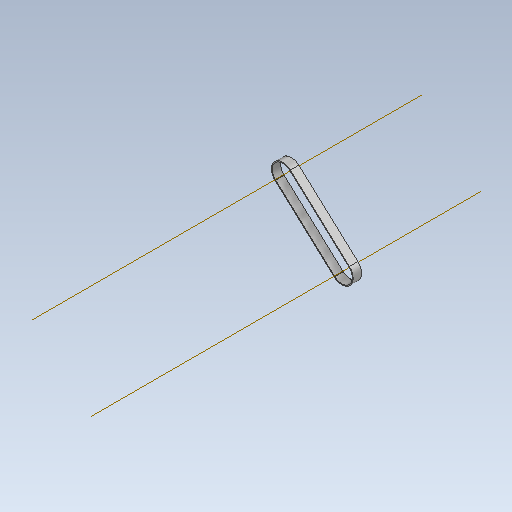
# Autodesk Inventor part: Synchronous Belt
Saved by Autodesk Inventor 2020 (Build 240168000, 168)
## iProperties
Created: 2022-07-06
Part Number: Synchronous Belt
Material: Rubber
Document SubType Name: Modeling
Designer: karimi2
Density: 1 g/cm^3
Appearance: Rubber - Black - Version 1.1
CustomPartVersion: 1
Author: karimi2
Autodesk Inventor part; units mm, degrees
sketch "Sketch Path" plane through (0, 0, 0) normal (0, 0, 1) x (1, 0, 0)
  arc A0 (-122.9906, 123.6577) -> (-133.8904, 111.7133) centre (-128.4405, 117.6855) ccw
  arc A1 (-89.5701, 71.2694) -> (-78.6704, 83.2138) centre (-84.1202, 77.2416) ccw
  line L0 (-89.5701, 71.2694) -> (-133.8904, 111.7133)
  line L1 (-122.9906, 123.6577) -> (-78.6704, 83.2138)
  constraints: 4 end point, 4 point on circle, 2 centre point
ref_plane "Cross Section Plane" through (-133.8904, 111.7133, 0) normal (0.7387, -0.6741, 0) x (0, 0, 1)
ref_plane "Work Plane2" through (-128.4405, 117.6855, 0) normal (-1, 0, 0) x (0, 0, 1)
ref_plane "Work Plane3" through (-84.1202, 77.2416, 0) normal (-0.6427, 0.7661, 0) x (0, 0, 1)
sketch "Cross Section" plane through (-133.8904, 111.7133, 0) normal (0.7387, -0.6741, 0) x (0, 0, 1)
  line L0 (-3.175, 0.381) -> (3.175, 0.381)
  line L1 (3.175, 0.381) -> (3.175, -0.254)
  line L2 (3.175, -0.254) -> (-3.175, -0.254)
  line L3 (-3.175, -0.254) -> (-3.175, 0.381)
  line L4 (-3.175, 0) -> (3.175, 0) construction
  point P0 (0, 0)
  point P1 (0, 0)
  dimension "d0" = 6.35
  dimension "d4" = 0.254
  dimension "d5" = 0.381
  constraints: 10 end point, 2 parallel, 2 point on line, 1 coincident, 1 horizontal, 1 midpoint, 1 perpendicular, 1 other
  measures "d0" distance between parallel lines of L1 L3
  measures "d4" distance between parallel lines of L2 L4
  measures "d5" distance between parallel lines of L4 L0
sweep "Belt" add profiles "Cross Section" path "Sketch Path"
equation "\"d0\" = da_B"
equation "\"d4\" = da_a"
equation "\"d5\" = da_a2"
equation "\"da_B\" = 6.35"
equation "\"da_pb\" = 2.032"
equation "\"da_L\" = 170.8"
equation "\"da_a\" = 0.254"
equation "\"da_S\" = 1.143"
equation "\"da_Beta\" = 20deg"
equation "\"da_Ht\" = 0.508"
equation "\"da_H\" = 1.143"
equation "\"da_a2\" = 0.381"
body "Solid1"
